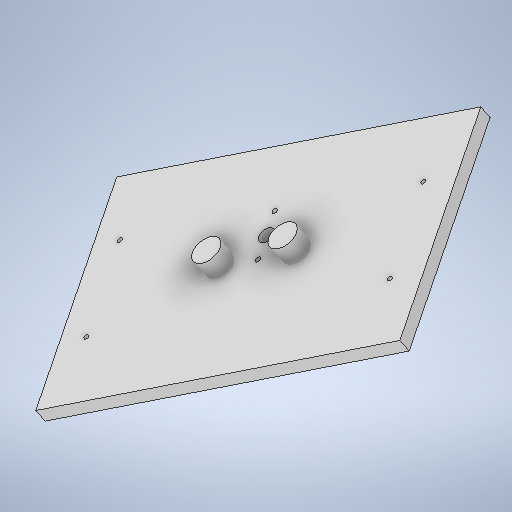
# Autodesk Inventor part: Grundplatte_v4
Saved by Autodesk Inventor 2025 (Build 290162000, 162)
## iProperties
Created: 2026-07-10
Part Number: Grundplatte_v4
Material: Generisch
Document SubType Name: Modeling
Designer: wavid
Mass: 242.026 g
Surface Area: 678.708 cm^2
Volume: 242.026 cm^3
Density: 1 g/cm^3
Appearance: Vorgabe
Author: wavid
Autodesk Inventor part; units mm, degrees
ref_plane "YZ Plane" through (0, 0, 0) normal (1, 0, 0) x (0, 1, 0)
ref_plane "XZ Plane" through (0, 0, 0) normal (0, 1, 0) x (-1, 0, 0)
sketch "Skizze1" plane through (0, 0, 0) normal (0, 0, 1) x (1, 0, 0)
  line L0 (-70, -105) -> (70, -105)
  line L1 (70, -105) -> (70, 105)
  line L2 (70, 105) -> (-70, 105)
  line L3 (-70, 105) -> (-70, -105)
  constraints: 8 end point, 2 parallel, 1 horizontal, 1 perpendicular
extrude "Extrusion1" add sketch "Skizze1" along normal blind 8
ref_plane "Arbeitsebene1" through (0, 0, 8) normal (0, 0, 1) x (1, 0, 0)
sketch "Skizze2" plane through (0, 0, 8) normal (0, 0, 1) x (1, 0, 0)
  circle A0 centre (-14, 0) radius 4.5
  constraints: 1 centre point
extrude "Extrusion2" cut sketch "Skizze2" against normal blind 8.2
sketch "Skizze3" plane through (0, 0, 8) normal (0, 0, 1) x (1, 0, 0)
  circle A0 centre (-28.5, 0) radius 1.6
  constraints: 1 centre point
extrude "Extrusion3" cut sketch "Skizze3" against normal blind 8.2
sketch "Skizze4" plane through (0, 0, 8) normal (0, 0, 1) x (1, 0, 0)
  circle A0 centre (0.5, 0) radius 1.6
  constraints: 1 centre point
extrude "Extrusion4" cut sketch "Skizze4" against normal blind 8.2
sketch "Skizze5" plane through (0, 0, 8) normal (0, 0, 1) x (1, 0, 0)
  circle A0 centre (-29, -89.5) radius 1.4
  constraints: 1 centre point
extrude "Extrusion5" cut sketch "Skizze5" against normal blind 8.2
sketch "Skizze6" plane through (0, 0, 8) normal (0, 0, 1) x (1, 0, 0)
  circle A0 centre (29, -89.5) radius 1.4
  constraints: 1 centre point
extrude "Extrusion6" cut sketch "Skizze6" against normal blind 8.2
sketch "Skizze7" plane through (0, 0, 8) normal (0, 0, 1) x (1, 0, 0)
  circle A0 centre (-29, 85.5) radius 1.4
  constraints: 1 centre point
extrude "Extrusion7" cut sketch "Skizze7" against normal blind 8.2
sketch "Skizze8" plane through (0, 0, 8) normal (0, 0, 1) x (1, 0, 0)
  circle A0 centre (29, 85.5) radius 1.4
  constraints: 1 centre point
extrude "Extrusion8" cut sketch "Skizze8" against normal blind 8.2
sketch "Skizze9" plane through (0, 0, 0) normal (0, 0, 1) x (1, 0, 0)
  circle A0 centre (0, -22) radius 8
  constraints: 1 centre point
extrude "Extrusion9" add sketch "Skizze9" along normal blind 20 separate body
sketch "Skizze10" plane through (0, 0, 0) normal (0, 0, 1) x (1, 0, 0)
  circle A0 centre (0, 22) radius 8
  constraints: 1 centre point
extrude "Extrusion10" add sketch "Skizze10" along normal blind 20 separate body
ref_plane "Arbeitsebene2" through (0, 0, 20) normal (0, 0, 1) x (1, 0, 0)
sketch "Skizze11" plane through (0, 0, 20) normal (0, 0, 1) x (1, 0, 0)
  circle A0 centre (0, -22) radius 3.9
  constraints: 1 centre point
extrude "Extrusion11" cut sketch "Skizze11" against normal blind 16 bodies 1
sketch "Skizze12" plane through (0, 0, 20) normal (0, 0, 1) x (1, 0, 0)
  circle A0 centre (0, 22) radius 3.9
  constraints: 1 centre point
extrude "Extrusion12" cut sketch "Skizze12" against normal blind 16 bodies 1
